Autodesk Inventor part; units mm, degrees
(part 14 of 15)
  line L310 (15.292, -114.284) -> (15.292, -116.316)
  line L311 (15.292, -116.316) -> (16.308, -116.316)
  line L312 (3.408, 49.384) -> (3.408, 51.416)
  line L313 (10.057, -106.5108) -> (10.057, -111.4892)
  line L314 (10.057, -111.4892) -> (12.343, -111.4892)
  line L315 (12.343, -111.4892) -> (12.343, -106.5108)
  line L316 (12.343, -106.5108) -> (10.057, -106.5108)
  line L317 (3.408, 51.416) -> (2.392, 51.416)
  line L318 (1.457, -107.4108) -> (1.457, -112.3892)
  line L319 (1.457, -112.3892) -> (3.743, -112.3892)
  line L320 (3.743, -112.3892) -> (3.743, -107.4108)
  line L321 (3.743, -107.4108) -> (1.457, -107.4108)
  line L322 (2.392, 51.416) -> (2.392, 49.384)
  line L323 (3.765, -108.503) -> (3.765, -111.297)
  line L324 (3.765, -111.297) -> (5.035, -111.297)
  line L325 (5.035, -111.297) -> (5.035, -108.503)
  line L326 (5.035, -108.503) -> (3.765, -108.503)
  line L327 (2.392, 49.384) -> (3.408, 49.384)
  line L328 (8.765, -108.503) -> (8.765, -111.297)
  line L329 (8.765, -111.297) -> (10.035, -111.297)
  line L330 (10.035, -111.297) -> (10.035, -108.503)
  line L331 (10.035, -108.503) -> (8.765, -108.503)
  line L332 (8.616, 35.608) -> (6.584, 35.608)
  line L333 (11.824, -116.313) -> (11.824, -111.487)
  line L334 (11.824, -111.487) -> (8.776, -111.487)
  line L335 (8.776, -111.487) -> (8.776, -116.313)
  line L336 (8.776, -116.313) -> (11.824, -116.313)
  line L337 (6.584, 35.608) -> (6.584, 34.592)
  line L338 (3.776, -100.887) -> (3.776, -105.713)
  line L339 (3.776, -105.713) -> (6.824, -105.713)
  line L340 (6.824, -105.713) -> (6.824, -100.887)
  line L341 (6.824, -100.887) -> (3.776, -100.887)
  line L342 (6.584, 34.592) -> (8.616, 34.592)
  line L343 (16.403, -99.635) -> (19.197, -99.635)
  line L344 (19.197, -99.635) -> (19.197, -98.365)
  line L345 (19.197, -98.365) -> (16.403, -98.365)
  line L346 (16.403, -98.365) -> (16.403, -99.635)
  line L347 (8.616, 34.592) -> (8.616, 35.608)
  line L348 (8.765, -100.903) -> (8.765, -103.697)
  line L349 (8.765, -103.697) -> (10.035, -103.697)
  line L350 (10.035, -103.697) -> (10.035, -100.903)
  line L351 (10.035, -100.903) -> (8.765, -100.903)
  line L352 (8.584, 43.992) -> (10.616, 43.992)
  line L353 (7.165, -100.903) -> (7.165, -103.697)
  line L354 (7.165, -103.697) -> (8.435, -103.697)
  line L355 (8.435, -103.697) -> (8.435, -100.903)
  line L356 (8.435, -100.903) -> (7.165, -100.903)
  line L357 (10.616, 43.992) -> (10.616, 45.008)
  line L358 (-7.387, -104.576) -> (-12.213, -104.576)
  line L359 (-12.213, -104.576) -> (-12.213, -107.624)
  line L360 (-12.213, -107.624) -> (-7.387, -107.624)
  line L361 (-7.387, -107.624) -> (-7.387, -104.576)
  line L362 (10.616, 45.008) -> (8.584, 45.008)
  line L363 (-9.403, -107.965) -> (-12.197, -107.965)
  line L364 (-12.197, -107.965) -> (-12.197, -109.235)
  line L365 (-12.197, -109.235) -> (-9.403, -109.235)
  line L366 (-9.403, -109.235) -> (-9.403, -107.965)
  line L367 (8.584, 45.008) -> (8.584, 43.992)
  line L368 (-4.916, -113.308) -> (-2.884, -113.308)
  line L369 (-2.884, -113.308) -> (-2.884, -112.292)
  line L370 (-2.884, -112.292) -> (-4.916, -112.292)
  line L371 (-4.916, -112.292) -> (-4.916, -113.308)
  line L372 (7.592, 37.616) -> (7.592, 35.584)
  line L373 (11.184, -98.108) -> (13.216, -98.108)
  line L374 (13.216, -98.108) -> (13.216, -97.092)
  line L375 (13.216, -97.092) -> (11.184, -97.092)
  line L376 (11.184, -97.092) -> (11.184, -98.108)
  line L377 (7.592, 35.584) -> (8.608, 35.584)
  line L378 (-7.784, -111.692) -> (-9.816, -111.692)
  line L379 (-9.816, -111.692) -> (-9.816, -112.708)
  line L380 (-9.816, -112.708) -> (-7.784, -112.708)
  line L381 (-7.784, -112.708) -> (-7.784, -111.692)
  line L382 (8.608, 35.584) -> (8.608, 37.616)
  line L383 (17.765, -99.803) -> (17.765, -102.597)
  line L384 (17.765, -102.597) -> (19.035, -102.597)
  line L385 (19.035, -102.597) -> (19.035, -99.803)
  line L386 (19.035, -99.803) -> (17.765, -99.803)
  line L387 (8.608, 37.616) -> (7.592, 37.616)
  line L388 (16.465, -99.803) -> (16.465, -102.597)
  line L389 (16.465, -102.597) -> (17.735, -102.597)
  line L390 (17.735, -102.597) -> (17.735, -99.803)
  line L391 (17.735, -99.803) -> (16.465, -99.803)
  line L392 (7.608, 35.584) -> (7.608, 37.616)
  line L393 (-2.892, -111.316) -> (-2.892, -109.284)
  line L394 (-2.892, -109.284) -> (-3.908, -109.284)
  line L395 (-3.908, -109.284) -> (-3.908, -111.316)
  line L396 (-3.908, -111.316) -> (-2.892, -111.316)
  line L397 (7.608, 37.616) -> (6.592, 37.616)
  line L398 (-9.676, -117.913) -> (-9.676, -113.087)
  line L399 (-9.676, -113.087) -> (-12.724, -113.087)
  line L400 (-12.724, -113.087) -> (-12.724, -117.913)
  line L401 (-12.724, -117.913) -> (-9.676, -117.913)
  line L402 (6.592, 37.616) -> (6.592, 35.584)
  line L403 (3.776, -94.687) -> (3.776, -99.513)
  line L404 (3.776, -99.513) -> (6.824, -99.513)
  line L405 (6.824, -99.513) -> (6.824, -94.687)
  line L406 (6.824, -94.687) -> (3.776, -94.687)
  line L407 (6.592, 35.584) -> (7.608, 35.584)
  line L408 (-8.5892, 45.257) -> (-3.6108, 45.257)
  line L409 (-3.6108, 45.257) -> (-3.6108, 47.543)
  line L410 (-3.6108, 47.543) -> (-8.5892, 47.543)
  line L411 (-8.5892, 47.543) -> (-8.5892, 45.257)
  line L412 (8.608, 45.984) -> (8.608, 48.016)
  line L413 (-9.2892, 36.757) -> (-4.3108, 36.757)
  line L414 (-4.3108, 36.757) -> (-4.3108, 39.043)
  line L415 (-4.3108, 39.043) -> (-9.2892, 39.043)
  line L416 (-9.2892, 39.043) -> (-9.2892, 36.757)
  line L417 (8.608, 48.016) -> (7.592, 48.016)
  line L418 (-4.343, 43.6892) -> (-4.343, 38.7108)
  line L419 (-4.343, 38.7108) -> (-2.057, 38.7108)
  line L420 (-2.057, 38.7108) -> (-2.057, 43.6892)
  line L421 (-2.057, 43.6892) -> (-4.343, 43.6892)
  line L422 (7.592, 48.016) -> (7.592, 45.984)
  line L423 (-6.616, 44.292) -> (-4.584, 44.292)
  line L424 (-4.584, 44.292) -> (-4.584, 45.308)
  line L425 (-4.584, 45.308) -> (-6.616, 45.308)
  line L426 (-6.616, 45.308) -> (-6.616, 44.292)
  line L427 (7.592, 45.984) -> (8.608, 45.984)
  line L428 (0.1542, 45.489) -> (-3.5542, 45.489)
  line L429 (-3.5542, 45.489) -> (-3.5542, 43.711)
  line L430 (-3.5542, 43.711) -> (0.1542, 43.711)
  line L431 (0.1542, 43.711) -> (0.1542, 45.489)
  line L432 (2.308, 43.784) -> (2.308, 45.816)
  line L433 (-2.311, 34.9458) -> (-2.311, 38.6542)
  line L434 (-2.311, 38.6542) -> (-4.089, 38.6542)
  line L435 (-4.089, 38.6542) -> (-4.089, 34.9458)
  line L436 (-4.089, 34.9458) -> (-2.311, 34.9458)
  line L437 (2.308, 45.816) -> (1.292, 45.816)
  line L438 (-3.589, 49.2542) -> (-3.589, 45.5458)
  line L439 (-3.589, 45.5458) -> (-1.811, 45.5458)
  line L440 (-1.811, 45.5458) -> (-1.811, 49.2542)
  line L441 (-1.811, 49.2542) -> (-3.589, 49.2542)
  line L442 (1.292, 45.816) -> (1.292, 43.784)
  line L443 (2.916, -93.492) -> (0.884, -93.492)
  line L444 (0.884, -93.492) -> (0.884, -94.508)
  line L445 (0.884, -94.508) -> (2.916, -94.508)
  line L446 (2.916, -94.508) -> (2.916, -93.492)
  line L447 (1.292, 43.784) -> (2.308, 43.784)
  line L448 (-23.584, -18.692) -> (-25.616, -18.692)
  line L449 (-25.616, -18.692) -> (-25.616, -19.708)
  line L450 (-25.616, -19.708) -> (-23.584, -19.708)
  line L451 (-23.584, -19.708) -> (-23.584, -18.692)
  line L452 (4.316, 44.808) -> (2.284, 44.808)
  line L453 (-23.584, -15.692) -> (-25.616, -15.692)
  line L454 (-25.616, -15.692) -> (-25.616, -16.708)
  line L455 (-25.616, -16.708) -> (-23.584, -16.708)
  line L456 (-23.584, -16.708) -> (-23.584, -15.692)
  line L457 (2.284, 44.808) -> (2.284, 43.792)
  line L458 (-25.608, -16.684) -> (-25.608, -18.716)
  line L459 (-25.608, -18.716) -> (-24.592, -18.716)
  line L460 (-24.592, -18.716) -> (-24.592, -16.684)
  line L461 (-24.592, -16.684) -> (-25.608, -16.684)
  line L462 (2.284, 43.792) -> (4.316, 43.792)
  line L463 (-19.784, -25.192) -> (-21.816, -25.192)
  line L464 (-21.816, -25.192) -> (-21.816, -26.208)
  line L465 (-21.816, -26.208) -> (-19.784, -26.208)
  line L466 (-19.784, -26.208) -> (-19.784, -25.192)
  line L467 (4.316, 43.792) -> (4.316, 44.808)
  line L468 (-22.184, -22.392) -> (-24.216, -22.392)
  line L469 (-24.216, -22.392) -> (-24.216, -23.408)
  line L470 (-24.216, -23.408) -> (-22.184, -23.408)
  line L471 (-22.184, -23.408) -> (-22.184, -22.392)
  line L472 (3.316, 47.008) -> (1.284, 47.008)
  line L473 (-21.808, -19.984) -> (-21.808, -22.016)
  line L474 (-21.808, -22.016) -> (-20.792, -22.016)
  line L475 (-20.792, -22.016) -> (-20.792, -19.984)
  line L476 (-20.792, -19.984) -> (-21.808, -19.984)
  line L477 (1.284, 47.008) -> (1.284, 45.992)
  line L478 (-1.784, -16.092) -> (-3.816, -16.092)
  line L479 (-3.816, -16.092) -> (-3.816, -17.108)
  line L480 (-3.816, -17.108) -> (-1.784, -17.108)
  line L481 (-1.784, -17.108) -> (-1.784, -16.092)
  line L482 (1.284, 45.992) -> (3.316, 45.992)
  line L483 (-7.216, -22.108) -> (-5.184, -22.108)
  line L484 (-5.184, -22.108) -> (-5.184, -21.092)
  line L485 (-5.184, -21.092) -> (-7.216, -21.092)
  line L486 (-7.216, -21.092) -> (-7.216, -22.108)
  line L487 (3.316, 45.992) -> (3.316, 47.008)
  line L488 (-1.784, -15.092) -> (-3.816, -15.092)
  line L489 (-3.816, -15.092) -> (-3.816, -16.108)
  line L490 (-3.816, -16.108) -> (-1.784, -16.108)
  line L491 (-1.784, -16.108) -> (-1.784, -15.092)
  line L492 (1.284, 46.992) -> (3.316, 46.992)
  line L493 (-7.216, -20.108) -> (-5.184, -20.108)
  line L494 (-5.184, -20.108) -> (-5.184, -19.092)
  line L495 (-5.184, -19.092) -> (-7.216, -19.092)
  line L496 (-7.216, -19.092) -> (-7.216, -20.108)
  line L497 (3.316, 46.992) -> (3.316, 48.008)
  line L498 (-7.216, -19.108) -> (-5.184, -19.108)
  line L499 (-5.184, -19.108) -> (-5.184, -18.092)
  line L500 (-5.184, -18.092) -> (-7.216, -18.092)
  line L501 (-7.216, -18.092) -> (-7.216, -19.108)
  line L502 (3.316, 48.008) -> (1.284, 48.008)
  line L503 (-7.216, -17.108) -> (-5.184, -17.108)
  line L504 (-5.184, -17.108) -> (-5.184, -16.092)
  line L505 (-5.184, -16.092) -> (-7.216, -16.092)
  line L506 (-7.216, -16.092) -> (-7.216, -17.108)
  line L507 (1.284, 48.008) -> (1.284, 46.992)
  line L508 (-1.784, -18.092) -> (-3.816, -18.092)
  line L509 (-3.816, -18.092) -> (-3.816, -19.108)
  line L510 (-3.816, -19.108) -> (-1.784, -19.108)
  line L511 (-1.784, -19.108) -> (-1.784, -18.092)
  line L512 (4.316, 39.808) -> (2.284, 39.808)
  line L513 (-7.216, -16.108) -> (-5.184, -16.108)
  line L514 (-5.184, -16.108) -> (-5.184, -15.092)
  line L515 (-5.184, -15.092) -> (-7.216, -15.092)
  line L516 (-7.216, -15.092) -> (-7.216, -16.108)
  line L517 (2.284, 39.808) -> (2.284, 38.792)
  line L518 (-7.216, -23.108) -> (-5.184, -23.108)
  line L519 (-5.184, -23.108) -> (-5.184, -22.092)
  line L520 (-5.184, -22.092) -> (-7.216, -22.092)
  line L521 (-7.216, -22.092) -> (-7.216, -23.108)
  line L522 (2.284, 38.792) -> (4.316, 38.792)
  line L523 (-1.784, -21.092) -> (-3.816, -21.092)
  line L524 (-3.816, -21.092) -> (-3.816, -22.108)
  line L525 (-3.816, -22.108) -> (-1.784, -22.108)
  line L526 (-1.784, -22.108) -> (-1.784, -21.092)
  line L527 (4.316, 38.792) -> (4.316, 39.808)
  line L528 (-1.784, -22.092) -> (-3.816, -22.092)
  line L529 (-3.816, -22.092) -> (-3.816, -23.108)
  line L530 (-3.816, -23.108) -> (-1.784, -23.108)
  line L531 (-1.784, -23.108) -> (-1.784, -22.092)
  line L532 (17.084, -58.708) -> (19.116, -58.708)
  line L533 (-1.784, -19.092) -> (-3.816, -19.092)
  line L534 (-3.816, -19.092) -> (-3.816, -20.108)
  line L535 (-3.816, -20.108) -> (-1.784, -20.108)
  line L536 (-1.784, -20.108) -> (-1.784, -19.092)
  line L537 (19.116, -58.708) -> (19.116, -57.692)
  line L538 (-7.216, -24.108) -> (-5.184, -24.108)
  line L539 (-5.184, -24.108) -> (-5.184, -23.092)
  line L540 (-5.184, -23.092) -> (-7.216, -23.092)
  line L541 (-7.216, -23.092) -> (-7.216, -24.108)
  line L542 (19.116, -57.692) -> (17.084, -57.692)
  line L543 (2.308, -40.816) -> (2.308, -38.784)
  line L544 (2.308, -38.784) -> (1.292, -38.784)
  line L545 (1.292, -38.784) -> (1.292, -40.816)
  line L546 (1.292, -40.816) -> (2.308, -40.816)
  line L547 (17.084, -57.692) -> (17.084, -58.708)
  line L548 (2.284, -38.808) -> (4.316, -38.808)
  line L549 (4.316, -38.808) -> (4.316, -37.792)
  line L550 (4.316, -37.792) -> (2.284, -37.792)
  line L551 (2.284, -37.792) -> (2.284, -38.808)
  line L552 (20.184, -54.908) -> (22.216, -54.908)
  line L553 (-14.316, -41.608) -> (-12.284, -41.608)
  line L554 (-12.284, -41.608) -> (-12.284, -40.592)
  line L555 (-12.284, -40.592) -> (-14.316, -40.592)
  line L556 (-14.316, -40.592) -> (-14.316, -41.608)
  line L557 (22.216, -54.908) -> (22.216, -53.892)
  line L558 (6.208, -40.816) -> (6.208, -38.784)
  line L559 (6.208, -38.784) -> (5.192, -38.784)
  line L560 (5.192, -38.784) -> (5.192, -40.816)
  line L561 (5.192, -40.816) -> (6.208, -40.816)
  line L562 (22.216, -53.892) -> (20.184, -53.892)
  line L563 (6.184, -38.808) -> (8.216, -38.808)
  line L564 (8.216, -38.808) -> (8.216, -37.792)
  line L565 (8.216, -37.792) -> (6.184, -37.792)
  line L566 (6.184, -37.792) -> (6.184, -38.808)
  line L567 (20.184, -53.892) -> (20.184, -54.908)
  line L568 (-5.092, -42.516) -> (-5.092, -40.484)
  line L569 (-5.092, -40.484) -> (-6.108, -40.484)
  line L570 (-6.108, -40.484) -> (-6.108, -42.516)
  line L571 (-6.108, -42.516) -> (-5.092, -42.516)
  line L572 (20.184, -55.908) -> (22.216, -55.908)
  line L573 (21.908, -43.516) -> (21.908, -41.484)
  line L574 (21.908, -41.484) -> (20.892, -41.484)
  line L575 (20.892, -41.484) -> (20.892, -43.516)
  line L576 (20.892, -43.516) -> (21.908, -43.516)
  line L577 (22.216, -55.908) -> (22.216, -54.892)
  line L578 (13.184, -46.208) -> (15.216, -46.208)
  line L579 (15.216, -46.208) -> (15.216, -45.192)
  line L580 (15.216, -45.192) -> (13.184, -45.192)
  line L581 (13.184, -45.192) -> (13.184, -46.208)
  line L582 (22.216, -54.892) -> (20.184, -54.892)
  line L583 (14.092, -48.284) -> (14.092, -50.316)
  line L584 (14.092, -50.316) -> (15.108, -50.316)
  line L585 (15.108, -50.316) -> (15.108, -48.284)
  line L586 (15.108, -48.284) -> (14.092, -48.284)
  line L587 (20.184, -54.892) -> (20.184, -55.908)
  line L588 (17.808, -50.316) -> (17.808, -48.284)
  line L589 (17.808, -48.284) -> (16.792, -48.284)
  line L590 (16.792, -48.284) -> (16.792, -50.316)
  line L591 (16.792, -50.316) -> (17.808, -50.316)
  line L592 (20.184, -56.908) -> (22.216, -56.908)
  line L593 (13.184, -47.208) -> (15.216, -47.208)
  line L594 (15.216, -47.208) -> (15.216, -46.192)
  line L595 (15.216, -46.192) -> (13.184, -46.192)
  line L596 (13.184, -46.192) -> (13.184, -47.208)
  line L597 (22.216, -56.908) -> (22.216, -55.892)
  line L598 (17.216, -46.192) -> (15.184, -46.192)
  line L599 (15.184, -46.192) -> (15.184, -47.208)
  line L600 (15.184, -47.208) -> (17.216, -47.208)
  line L601 (17.216, -47.208) -> (17.216, -46.192)
  line L602 (22.216, -55.892) -> (20.184, -55.892)
  line L603 (4.992, -54.784) -> (4.992, -56.816)
  line L604 (4.992, -56.816) -> (6.008, -56.816)
  line L605 (6.008, -56.816) -> (6.008, -54.784)
  line L606 (6.008, -54.784) -> (4.992, -54.784)
  line L607 (20.184, -55.892) -> (20.184, -56.908)
  line L608 (-3.084, -51.692) -> (-5.116, -51.692)
  line L609 (-5.116, -51.692) -> (-5.116, -52.708)
  line L610 (-5.116, -52.708) -> (-3.084, -52.708)
  line L611 (-3.084, -52.708) -> (-3.084, -51.692)
  line L612 (20.184, -57.908) -> (22.216, -57.908)
  line L613 (-3.084, -48.692) -> (-5.116, -48.692)
  line L614 (-5.116, -48.692) -> (-5.116, -49.708)
  line L615 (-5.116, -49.708) -> (-3.084, -49.708)
  line L616 (-3.084, -49.708) -> (-3.084, -48.692)
  line L617 (22.216, -57.908) -> (22.216, -56.892)
  line L618 (-3.084, -45.692) -> (-5.116, -45.692)
  line L619 (-5.116, -45.692) -> (-5.116, -46.708)
  line L620 (-5.116, -46.708) -> (-3.084, -46.708)
  line L621 (-3.084, -46.708) -> (-3.084, -45.692)
  line L622 (22.216, -56.892) -> (20.184, -56.892)
  line L623 (-3.084, -42.692) -> (-5.116, -42.692)
  line L624 (-5.116, -42.692) -> (-5.116, -43.708)
  line L625 (-5.116, -43.708) -> (-3.084, -43.708)
  line L626 (-3.084, -43.708) -> (-3.084, -42.692)
  line L627 (20.184, -56.892) -> (20.184, -57.908)
  line L628 (5.384, 52.492) -> (7.416, 52.492)
  line L629 (7.416, 52.492) -> (7.416, 53.508)
  line L630 (7.416, 53.508) -> (5.384, 53.508)
  line L631 (5.384, 53.508) -> (5.384, 52.492)
  line L632 (25.316, -56.492) -> (23.284, -56.492)
  line L633 (5.384, 53.492) -> (7.416, 53.492)
  line L634 (7.416, 53.492) -> (7.416, 54.508)
  line L635 (7.416, 54.508) -> (5.384, 54.508)
  line L636 (5.384, 54.508) -> (5.384, 53.492)
  line L637 (23.284, -56.492) -> (23.284, -57.508)
  line L638 (-0.684, 59.708) -> (-2.716, 59.708)
  line L639 (-2.716, 59.708) -> (-2.716, 58.692)
  line L640 (-2.716, 58.692) -> (-0.684, 58.692)
  line L641 (-0.684, 58.692) -> (-0.684, 59.708)
  line L642 (23.284, -57.508) -> (25.316, -57.508)
  line L643 (4.603, 54.565) -> (7.397, 54.565)
  line L644 (7.397, 54.565) -> (7.397, 55.835)
  line L645 (7.397, 55.835) -> (4.603, 55.835)
  line L646 (4.603, 55.835) -> (4.603, 54.565)
  line L647 (25.316, -57.508) -> (25.316, -56.492)
  line L648 (-0.697, 57.665) -> (2.097, 57.665)
  line L649 (2.097, 57.665) -> (2.097, 58.935)
  line L650 (2.097, 58.935) -> (-0.697, 58.935)
  line L651 (-0.697, 58.935) -> (-0.697, 57.665)
  line L652 (25.316, -57.492) -> (23.284, -57.492)
  line L653 (1.616, 54.308) -> (-0.416, 54.308)
  line L654 (-0.416, 54.308) -> (-0.416, 53.292)
  line L655 (-0.416, 53.292) -> (1.616, 53.292)
  line L656 (1.616, 53.292) -> (1.616, 54.308)
  line L657 (23.284, -57.492) -> (23.284, -58.508)
  line L658 (1.616, 53.308) -> (-0.416, 53.308)
  line L659 (-0.416, 53.308) -> (-0.416, 52.292)
  line L660 (-0.416, 52.292) -> (1.616, 52.292)
  line L661 (1.616, 52.292) -> (1.616, 53.308)
  line L662 (23.284, -58.508) -> (25.316, -58.508)
  line L663 (2.397, 52.235) -> (-0.397, 52.235)
  line L664 (-0.397, 52.235) -> (-0.397, 50.965)
  line L665 (-0.397, 50.965) -> (2.397, 50.965)
  line L666 (2.397, 50.965) -> (2.397, 52.235)
  line L667 (25.316, -58.508) -> (25.316, -57.492)
  line L668 (1.616, 57.708) -> (-0.416, 57.708)
  line L669 (-0.416, 57.708) -> (-0.416, 56.692)
  line L670 (-0.416, 56.692) -> (1.616, 56.692)
  line L671 (1.616, 56.692) -> (1.616, 57.708)
  line L672 (41.116, 51.508) -> (39.084, 51.508)
  line L673 (1.616, 56.708) -> (-0.416, 56.708)
  line L674 (-0.416, 56.708) -> (-0.416, 55.692)
  line L675 (-0.416, 55.692) -> (1.616, 55.692)
  line L676 (1.616, 55.692) -> (1.616, 56.708)
  line L677 (39.084, 51.508) -> (39.084, 50.492)
  line L678 (2.397, 55.635) -> (-0.397, 55.635)
  line L679 (-0.397, 55.635) -> (-0.397, 54.365)
  line L680 (-0.397, 54.365) -> (2.397, 54.365)
  line L681 (2.397, 54.365) -> (2.397, 55.635)
  line L682 (39.084, 50.492) -> (41.116, 50.492)
  line L683 (7.416, 51.508) -> (5.384, 51.508)
  line L684 (5.384, 51.508) -> (5.384, 50.492)
  line L685 (5.384, 50.492) -> (7.416, 50.492)
  line L686 (7.416, 50.492) -> (7.416, 51.508)
  line L687 (41.116, 50.492) -> (41.116, 51.508)
  line L688 (-0.584, 54.708) -> (-2.616, 54.708)
  line L689 (-2.616, 54.708) -> (-2.616, 53.692)
  line L690 (-2.616, 53.692) -> (-0.584, 53.692)
  line L691 (-0.584, 53.692) -> (-0.584, 54.708)
  line L692 (41.116, 50.508) -> (39.084, 50.508)
  line L693 (-0.584, 56.708) -> (-2.616, 56.708)
  line L694 (-2.616, 56.708) -> (-2.616, 55.692)
  line L695 (-2.616, 55.692) -> (-0.584, 55.692)
  line L696 (-0.584, 55.692) -> (-0.584, 56.708)
  line L697 (39.084, 50.508) -> (39.084, 49.492)
  line L698 (7.416, 52.508) -> (5.384, 52.508)
  line L699 (5.384, 52.508) -> (5.384, 51.492)
  line L700 (5.384, 51.492) -> (7.416, 51.492)
  line L701 (7.416, 51.492) -> (7.416, 52.508)
  line L702 (39.084, 49.492) -> (41.116, 49.492)
  line L703 (-0.584, 53.708) -> (-2.616, 53.708)
  line L704 (-2.616, 53.708) -> (-2.616, 52.692)
  line L705 (-2.616, 52.692) -> (-0.584, 52.692)
  line L706 (-0.584, 52.692) -> (-0.584, 53.708)
  line L707 (41.116, 49.492) -> (41.116, 50.508)
  line L708 (-0.584, 55.708) -> (-2.616, 55.708)
  line L709 (-2.616, 55.708) -> (-2.616, 54.692)
  line L710 (-2.616, 54.692) -> (-0.584, 54.692)
  line L711 (-0.584, 54.692) -> (-0.584, 55.708)
  line L712 (41.116, 49.508) -> (39.084, 49.508)
  line L713 (4.584, 34.592) -> (6.616, 34.592)
  line L714 (6.616, 34.592) -> (6.616, 35.608)
  line L715 (6.616, 35.608) -> (4.584, 35.608)
  line L716 (4.584, 35.608) -> (4.584, 34.592)
  line L717 (39.084, 49.508) -> (39.084, 48.492)
  line L718 (8.584, 42.992) -> (10.616, 42.992)
  line L719 (10.616, 42.992) -> (10.616, 44.008)
  line L720 (10.616, 44.008) -> (8.584, 44.008)
  line L721 (8.584, 44.008) -> (8.584, 42.992)
  line L722 (39.084, 48.492) -> (41.116, 48.492)
  line L723 (8.584, 41.992) -> (10.616, 41.992)
  line L724 (10.616, 41.992) -> (10.616, 43.008)
  line L725 (10.616, 43.008) -> (8.584, 43.008)
  line L726 (8.584, 43.008) -> (8.584, 41.992)
  line L727 (41.116, 48.492) -> (41.116, 49.508)
  line L728 (1.292, 43.816) -> (1.292, 41.784)
  line L729 (1.292, 41.784) -> (2.308, 41.784)
  line L730 (2.308, 41.784) -> (2.308, 43.816)
  line L731 (2.308, 43.816) -> (1.292, 43.816)
  line L732 (41.116, 48.508) -> (39.084, 48.508)
  line L733 (2.308, 39.784) -> (2.308, 41.816)
  line L734 (2.308, 41.816) -> (1.292, 41.816)
  line L735 (1.292, 41.816) -> (1.292, 39.784)
  line L736 (1.292, 39.784) -> (2.308, 39.784)
  line L737 (39.084, 48.508) -> (39.084, 47.492)
  line L738 (7.608, 45.984) -> (7.608, 48.016)
  line L739 (7.608, 48.016) -> (6.592, 48.016)
  line L740 (6.592, 48.016) -> (6.592, 45.984)
  line L741 (6.592, 45.984) -> (7.608, 45.984)
  line L742 (39.084, 47.492) -> (41.116, 47.492)
  line L743 (6.585, 46.003) -> (6.585, 48.797)
  line L744 (6.585, 48.797) -> (5.315, 48.797)
  line L745 (5.315, 48.797) -> (5.315, 46.003)
  line L746 (5.315, 46.003) -> (6.585, 46.003)
  line L747 (41.116, 47.492) -> (41.116, 48.508)
  line L748 (4.292, 48.016) -> (4.292, 45.984)
  line L749 (4.292, 45.984) -> (5.308, 45.984)
  line L750 (5.308, 45.984) -> (5.308, 48.016)
  line L751 (5.308, 48.016) -> (4.292, 48.016)
  line L752 (41.116, 44.008) -> (39.084, 44.008)
  line L753 (3.292, 48.016) -> (3.292, 45.984)
  line L754 (3.292, 45.984) -> (4.308, 45.984)
  line L755 (4.308, 45.984) -> (4.308, 48.016)
  line L756 (4.308, 48.016) -> (3.292, 48.016)
  line L757 (39.084, 44.008) -> (39.084, 42.992)
  line L758 (6.608, 35.584) -> (6.608, 37.616)
  line L759 (6.608, 37.616) -> (5.592, 37.616)
  line L760 (5.592, 37.616) -> (5.592, 35.584)
  line L761 (5.592, 35.584) -> (6.608, 35.584)
  line L762 (39.084, 42.992) -> (41.116, 42.992)
  line L763 (5.608, 35.584) -> (5.608, 37.616)
  line L764 (5.608, 37.616) -> (4.592, 37.616)
  line L765 (4.592, 37.616) -> (4.592, 35.584)
  line L766 (4.592, 35.584) -> (5.608, 35.584)
  line L767 (41.116, 42.992) -> (41.116, 44.008)
  line L768 (5.608, 37.584) -> (5.608, 39.616)
  line L769 (5.608, 39.616) -> (4.592, 39.616)
  line L770 (4.592, 39.616) -> (4.592, 37.584)
  line L771 (4.592, 37.584) -> (5.608, 37.584)
  line L772 (-23.116, -27.908) -> (-21.084, -27.908)
  line L773 (2.284, 42.792) -> (4.316, 42.792)
  line L774 (4.316, 42.792) -> (4.316, 43.808)
  line L775 (4.316, 43.808) -> (2.284, 43.808)
  line L776 (2.284, 43.808) -> (2.284, 42.792)
  line L777 (-21.084, -27.908) -> (-21.084, -26.892)
  line L778 (4.592, 46.016) -> (4.592, 43.984)
  line L779 (4.592, 43.984) -> (5.608, 43.984)
  line L780 (5.608, 43.984) -> (5.608, 46.016)
  line L781 (5.608, 46.016) -> (4.592, 46.016)
  line L782 (-21.084, -26.892) -> (-23.116, -26.892)
  line L783 (6.608, 37.584) -> (6.608, 39.616)
  line L784 (6.608, 39.616) -> (5.592, 39.616)
  line L785 (5.592, 39.616) -> (5.592, 37.584)
  line L786 (5.592, 37.584) -> (6.608, 37.584)
  line L787 (-23.116, -26.892) -> (-23.116, -27.908)
  line L788 (2.284, 41.792) -> (4.316, 41.792)
  line L789 (4.316, 41.792) -> (4.316, 42.808)
  line L790 (4.316, 42.808) -> (2.284, 42.808)
  line L791 (2.284, 42.808) -> (2.284, 41.792)
  line L792 (-23.284, -26.892) -> (-25.316, -26.892)
  line L793 (5.592, 46.016) -> (5.592, 43.984)
  line L794 (5.592, 43.984) -> (6.608, 43.984)
  line L795 (6.608, 43.984) -> (6.608, 46.016)
  line L796 (6.608, 46.016) -> (5.592, 46.016)
  line L797 (-25.316, -26.892) -> (-25.316, -27.908)
  line L798 (7.608, 37.584) -> (7.608, 39.616)
  line L799 (7.608, 39.616) -> (6.592, 39.616)
  line L800 (6.592, 39.616) -> (6.592, 37.584)
  line L801 (6.592, 37.584) -> (7.608, 37.584)
  line L802 (-25.316, -27.908) -> (-23.284, -27.908)
  line L803 (10.616, 41.608) -> (8.584, 41.608)
  line L804 (8.584, 41.608) -> (8.584, 40.592)
  line L805 (8.584, 40.592) -> (10.616, 40.592)
  line L806 (10.616, 40.592) -> (10.616, 41.608)
  line L807 (-23.284, -27.908) -> (-23.284, -26.892)
  line L808 (2.284, 40.792) -> (4.316, 40.792)
  line L809 (4.316, 40.792) -> (4.316, 41.808)
  line L810 (4.316, 41.808) -> (2.284, 41.808)
  line L811 (2.284, 41.808) -> (2.284, 40.792)
  line L812 (6.5, -90.25) -> (6.5, -91.34)
  line L813 (6.592, 46.016) -> (6.592, 43.984)
  line L814 (6.592, 43.984) -> (7.608, 43.984)
  line L815 (7.608, 43.984) -> (7.608, 46.016)
  line L816 (7.608, 46.016) -> (6.592, 46.016)
  line L817 (9.7, -90.05) -> (6.5, -90.05)
  line L818 (8.608, 37.584) -> (8.608, 39.616)
  line L819 (8.608, 39.616) -> (7.592, 39.616)
  line L820 (7.592, 39.616) -> (7.592, 37.584)
  line L821 (7.592, 37.584) -> (8.608, 37.584)
  line L822 (6.5, -90.05) -> (6.5, -91.55)
  line L823 (10.616, 40.608) -> (8.584, 40.608)
  line L824 (8.584, 40.608) -> (8.584, 39.592)
  line L825 (8.584, 39.592) -> (10.616, 39.592)
  line L826 (10.616, 39.592) -> (10.616, 40.608)
  line L827 (6.5, -91.55) -> (9.7, -91.55)
  line L828 (2.284, 39.792) -> (4.316, 39.792)
  line L829 (4.316, 39.792) -> (4.316, 40.808)
  line L830 (4.316, 40.808) -> (2.284, 40.808)
  line L831 (2.284, 40.808) -> (2.284, 39.792)
  line L832 (9.7, -91.55) -> (9.7, -90.05)
  line L833 (7.592, 46.016) -> (7.592, 43.984)
  line L834 (7.592, 43.984) -> (8.608, 43.984)
  line L835 (8.608, 43.984) -> (8.608, 46.016)
  line L836 (8.608, 46.016) -> (7.592, 46.016)
  circle A125 centre (9.29, -90.4) radius 0.15
  line L837 (18.608, -54.516) -> (18.608, -52.484)
  line L838 (18.608, -52.484) -> (17.592, -52.484)
  line L839 (17.592, -52.484) -> (17.592, -54.516)
  line L840 (17.592, -54.516) -> (18.608, -54.516)
  line L841 (2.05, -44.95) -> (5.15, -44.95)
  line L842 (23.284, -54.908) -> (25.316, -54.908)
  line L843 (25.316, -54.908) -> (25.316, -53.892)
  line L844 (25.316, -53.892) -> (23.284, -53.892)
  line L845 (23.284, -53.892) -> (23.284, -54.908)
  line L846 (5.15, -44.95) -> (5.15, -42.45)
  line L847 (-1.784, -20.092) -> (-3.816, -20.092)
  line L848 (-3.816, -20.092) -> (-3.816, -21.108)
  line L849 (-3.816, -21.108) -> (-1.784, -21.108)
  line L850 (-1.784, -21.108) -> (-1.784, -20.092)
  line L851 (5.15, -42.45) -> (2.05, -42.45)
  line L852 (-7.216, -18.108) -> (-5.184, -18.108)
  line L853 (-5.184, -18.108) -> (-5.184, -17.092)
  line L854 (-5.184, -17.092) -> (-7.216, -17.092)
  line L855 (-7.216, -17.092) -> (-7.216, -18.108)
  line L856 (2.05, -42.45) -> (2.05, -44.95)
  line L857 (-7.216, -21.108) -> (-5.184, -21.108)
  line L858 (-5.184, -21.108) -> (-5.184, -20.092)
  line L859 (-5.184, -20.092) -> (-7.216, -20.092)
  line L860 (-7.216, -20.092) -> (-7.216, -21.108)
  circle A126 centre (2.8, -43.1) radius 0.1
  line L861 (-1.784, -17.092) -> (-3.816, -17.092)
  line L862 (-3.816, -17.092) -> (-3.816, -18.108)
  line L863 (-3.816, -18.108) -> (-1.784, -18.108)
  line L864 (-1.784, -18.108) -> (-1.784, -17.092)
  line L865 (-20.584, -109.492) -> (-22.616, -109.492)
  line L866 (-22.616, -109.492) -> (-22.616, -110.508)
  line L867 (-22.616, -110.508) -> (-20.584, -110.508)
  line L868 (-20.584, -110.508) -> (-20.584, -109.492)
  line L869 (14.924, -116.313) -> (14.924, -111.487)
  line L870 (14.924, -111.487) -> (11.876, -111.487)
  line L871 (11.876, -111.487) -> (11.876, -116.313)
  line L872 (11.876, -116.313) -> (14.924, -116.313)
  line L873 (-47.3, -31.385) -> (-48.9, -31.385)
  circle A127 centre (-48.1, -47.7) radius 15.9
  line L874 (-16.5514, 47.555) -> (-16.5514, 47.255)
  line L875 (-16.5514, 46.455) -> (-16.5514, 46.155)
  line L876 (-16.5514, 45.355) -> (-16.5514, 45.055)
  line L877 (-16.5514, 44.255) -> (-16.5514, 43.955)
  line L878 (-16.5514, 43.155) -> (-16.5514, 42.855)
  line L879 (-16.5514, 42.055) -> (-16.5514, 41.755)
  line L880 (-16.5514, 40.955) -> (-16.5514, 40.655)
  line L881 (-16.5514, 39.855) -> (-16.5514, 39.555)
  line L882 (-22.4, 38.105) -> (-22.4, 37.385)
  line L883 (-15.05, 47.655) -> (-15.05, 39.105)
  arc A128 (-15.3, 38.855) -> (-15.05, 39.105) centre (-15.3, 39.105) ccw
  line L884 (-15.3, 38.855) -> (-16.3, 38.855)
  arc A129 (-16.55, 39.105) -> (-16.3, 38.855) centre (-16.3, 39.105) ccw
  line L885 (-16.55, 39.105) -> (-16.55, 47.655)
  arc A130 (-16.3, 47.905) -> (-16.55, 47.655) centre (-16.3, 47.655) ccw
  line L886 (-16.3, 47.905) -> (-15.3, 47.905)
  arc A131 (-15.05, 47.655) -> (-15.3, 47.905) centre (-15.3, 47.655) ccw
  line L887 (-24.45, 36.285) -> (-24.45, 36.105)
  line L888 (-24.45, 36.105) -> (-22.4, 36.105)
  line L889 (-22.4, 36.105) -> (-21.195, 36.105)
  line L890 (-21.195, 36.105) -> (-14.305, 36.105)
  line L891 (-14.305, 36.105) -> (-12.895, 36.105)
  line L892 (-12.895, 36.105) -> (-11.05, 36.105)
  line L893 (-11.05, 36.105) -> (-11.05, 37.155)
  line L894 (-11.05, 37.155) -> (-11.7948, 37.4261)
  arc A132 (-12.1166, 37.8115) -> (-11.7948, 37.4262) centre (-11.6238, 37.896) ccw
  arc A133 (-12.1167, 47.9985) -> (-12.1167, 37.8115) centre (17.6036, 42.905) ccw
  line L895 (-22.68, 36.295) -> (-25.5, 36.295)
  arc A134 (-25.55, 36.345) -> (-25.5, 36.295) centre (-25.5, 36.345) ccw
  line L896 (-25.55, 36.345) -> (-25.55, 36.805)
  arc A135 (-25.5, 36.855) -> (-25.55, 36.805) centre (-25.5, 36.805) ccw
  arc A136 (-25.55, 49.005) -> (-25.5, 48.955) centre (-25.5, 49.005) ccw
  line L897 (-25.55, 49.005) -> (-25.55, 49.465)
  arc A137 (-25.5, 49.515) -> (-25.55, 49.465) centre (-25.5, 49.465) ccw
  line L898 (-25.5, 49.515) -> (-22.68, 49.515)
  line L899 (-11.05, 48.655) -> (-11.05, 49.705)
  line L900 (-11.05, 49.705) -> (-12.895, 49.705)
  line L901 (-12.895, 49.705) -> (-14.305, 49.705)
  line L902 (-14.305, 49.705) -> (-21.195, 49.705)
  line L903 (-21.195, 49.705) -> (-22.4, 49.705)
  line L904 (-22.4, 49.705) -> (-24.45, 49.705)
  line L905 (-24.45, 49.705) -> (-24.45, 49.525)
  line L906 (-22.4, 36.105) -> (-22.4, 38.4841)
  line L907 (-22.4, 38.4841) -> (-22.4, 38.755)
  arc A138 (-22.4, 38.755) -> (-22.4, 38.955) centre (-22.4, 38.855) ccw
  line L908 (-22.4, 38.955) -> (-22.4, 39.305)
  arc A139 (-22.4, 39.305) -> (-22.4, 39.505) centre (-22.4, 39.405) ccw
  line L909 (-22.4, 39.505) -> (-22.4, 46.305)
  arc A140 (-22.4, 46.305) -> (-22.4, 46.505) centre (-22.4, 46.405) ccw
  line L910 (-22.4, 46.505) -> (-22.4, 46.855)
  arc A141 (-22.4, 46.855) -> (-22.4, 47.055) centre (-22.4, 46.955) ccw
  line L911 (-22.4, 47.055) -> (-22.4, 49.705)
  line L912 (-25.55, 38.4841) -> (-22.4, 38.4841)
  line L913 (-12.895, 49.705) -> (-12.895, 50.125)
  arc A142 (-12.895, 50.125) -> (-12.975, 50.205) centre (-12.975, 50.125) ccw
  line L914 (-12.975, 50.205) -> (-13.225, 50.205)
  line L915 (-13.225, 50.205) -> (-13.35, 50.085)
  line L916 (-13.35, 50.085) -> (-13.85, 50.085)
  line L917 (-13.85, 50.085) -> (-13.975, 50.205)
  line L918 (-13.975, 50.205) -> (-14.225, 50.205)
  arc A143 (-14.225, 50.205) -> (-14.305, 50.125) centre (-14.225, 50.125) ccw
  line L919 (-14.305, 50.125) -> (-14.305, 49.705)
  line L920 (-21.195, 49.705) -> (-21.195, 50.125)
  arc A144 (-21.195, 50.125) -> (-21.275, 50.205) centre (-21.275, 50.125) ccw
  line L921 (-21.275, 50.205) -> (-21.525, 50.205)
  line L922 (-21.525, 50.205) -> (-21.65, 50.085)
  line L923 (-21.65, 50.085) -> (-22.15, 50.085)
  line L924 (-22.15, 50.085) -> (-22.275, 50.205)
  line L925 (-22.275, 50.205) -> (-22.525, 50.205)
  arc A145 (-22.525, 50.205) -> (-22.605, 50.125) centre (-22.525, 50.125) ccw
  line L926 (-22.605, 50.125) -> (-22.605, 49.455)
  line L927 (-22.605, 49.455) -> (-22.6, 49.455)
  line L928 (-22.6, 49.455) -> (-22.6, 48.955)
  line L929 (-22.6, 48.955) -> (-23.1, 48.955)
  line L930 (-23.1, 48.955) -> (-23.1, 49.105)
  line L931 (-23.1, 49.105) -> (-22.85, 49.105)
  line L932 (-22.85, 49.105) -> (-22.8, 49.155)
  line L933 (-22.8, 49.155) -> (-22.8, 49.305)
  line L934 (-22.8, 49.305) -> (-22.85, 49.355)
  line L935 (-22.85, 49.355) -> (-25.3, 49.355)
  line L936 (-25.3, 49.355) -> (-25.35, 49.305)
  line L937 (-25.35, 49.305) -> (-25.35, 49.155)
  line L938 (-25.35, 49.155) -> (-25.3, 49.105)
  line L939 (-25.3, 49.105) -> (-25.05, 49.105)
  line L940 (-25.05, 49.105) -> (-25.05, 48.955)
  line L941 (-25.05, 48.955) -> (-25.55, 48.955)
  line L942 (-25.55, 48.955) -> (-25.55, 38.4841)
  line L943 (-25.55, 38.4841) -> (-25.55, 36.855)
  line L944 (-25.55, 36.855) -> (-25.05, 36.855)
  line L945 (-25.05, 36.855) -> (-25.05, 36.705)
  line L946 (-25.05, 36.705) -> (-25.3, 36.705)
  line L947 (-25.3, 36.705) -> (-25.35, 36.655)
  line L948 (-25.35, 36.655) -> (-25.35, 36.505)
  line L949 (-25.35, 36.505) -> (-25.3, 36.455)
  line L950 (-25.3, 36.455) -> (-22.85, 36.455)
  line L951 (-22.85, 36.455) -> (-22.8, 36.505)
  line L952 (-22.8, 36.505) -> (-22.8, 36.655)
  line L953 (-22.8, 36.655) -> (-22.85, 36.705)
  line L954 (-22.85, 36.705) -> (-23.1, 36.705)
  line L955 (-23.1, 36.705) -> (-23.1, 36.855)
  line L956 (-23.1, 36.855) -> (-22.6, 36.855)
  line L957 (-22.6, 36.855) -> (-22.6, 36.355)
  line L958 (-22.6, 36.355) -> (-22.605, 36.355)
  line L959 (-22.605, 36.355) -> (-22.605, 35.685)
  arc A146 (-22.605, 35.685) -> (-22.525, 35.605) centre (-22.525, 35.685) ccw
  line L960 (-22.525, 35.605) -> (-22.275, 35.605)
  line L961 (-22.275, 35.605) -> (-22.15, 35.725)
  line L962 (-22.15, 35.725) -> (-21.65, 35.725)
  line L963 (-21.65, 35.725) -> (-21.525, 35.605)
  line L964 (-21.525, 35.605) -> (-21.275, 35.605)
  arc A147 (-21.275, 35.605) -> (-21.195, 35.685) centre (-21.275, 35.685) ccw
  line L965 (-21.195, 35.685) -> (-21.195, 36.105)
  line L966 (-14.305, 36.105) -> (-14.305, 35.685)
  arc A148 (-14.305, 35.685) -> (-14.225, 35.605) centre (-14.225, 35.685) ccw
  line L967 (-14.225, 35.605) -> (-13.975, 35.605)
  line L968 (-13.975, 35.605) -> (-13.85, 35.725)
  line L969 (-13.85, 35.725) -> (-13.35, 35.725)
  line L970 (-13.35, 35.725) -> (-13.225, 35.605)
  line L971 (-13.225, 35.605) -> (-12.975, 35.605)
  arc A149 (-12.975, 35.605) -> (-12.895, 35.685) centre (-12.975, 35.685) ccw
  line L972 (-12.895, 35.685) -> (-12.895, 36.105)
  arc A150 (-11.7948, 48.3838) -> (-12.1166, 47.9985) centre (-11.6238, 47.914) ccw
  arc A151 (-11.7948, 48.3838) -> (-12.1166, 47.9985) centre (-11.6238, 47.914) ccw
  line L973 (-11.7948, 48.3839) -> (-11.05, 48.655)
  line L974 (65.55, 33.9) -> (70.05, 33.9)
  line L975 (70.05, 33.9) -> (70.05, 55.3)
  line L976 (70.05, 55.3) -> (65.55, 55.3)
  line L977 (65.55, 55.3) -> (65.55, 33.9)
  line L978 (66.3, 53.6) -> (67.3, 54.1)
  line L979 (66.3, 54.6) -> (66.3, 53.6)
  line L980 (67.3, 54.1) -> (66.3, 54.6)
  line L981 (22.55, -102.1) -> (25.05, -102.1)
  line L982 (25.05, -101.1) -> (22.55, -101.1)
  line L983 (25.05, -102.1) -> (25.05, -101.1)
  line L984 (22.55, -101.1) -> (22.55, -102.1)
  circle A152 centre (24.7, -101.8) radius 0.05
  line L985 (22.15, -101.1) -> (19.65, -101.1)
  line L986 (19.65, -102.1) -> (22.15, -102.1)
  line L987 (19.65, -101.1) -> (19.65, -102.1)
  line L988 (22.15, -102.1) -> (22.15, -101.1)
  circle A153 centre (20, -101.4) radius 0.05
  line L989 (-18.8, -16.95) -> (-18.8, -19.45)
  line L990 (-17.8, -19.45) -> (-17.8, -16.95)
  line L991 (-18.8, -19.45) -> (-17.8, -19.45)
  line L992 (-17.8, -16.95) -> (-18.8, -16.95)
  circle A154 centre (-18.5, -19.1) radius 0.05
  line L993 (-17.8, -16.65) -> (-17.8, -14.15)
  line L994 (-18.8, -14.15) -> (-18.8, -16.65)
  line L995 (-17.8, -14.15) -> (-18.8, -14.15)
  line L996 (-18.8, -16.65) -> (-17.8, -16.65)
  circle A155 centre (-18.1, -14.5) radius 0.05
  line L997 (22.05, -44.5) -> (19.55, -44.5)
  line L998 (19.55, -45.5) -> (22.05, -45.5)
  line L999 (19.55, -44.5) -> (19.55, -45.5)
  line L1000 (22.05, -45.5) -> (22.05, -44.5)
  circle A156 centre (19.9, -44.8) radius 0.05
  line L1001 (22.35, -45.5) -> (24.85, -45.5)
  line L1002 (24.85, -44.5) -> (22.35, -44.5)
  line L1003 (24.85, -45.5) -> (24.85, -44.5)
  line L1004 (22.35, -44.5) -> (22.35, -45.5)
  circle A157 centre (24.5, -45.2) radius 0.05
  line L1005 (0, -50.05) -> (0, -52.55)
  line L1006 (1, -52.55) -> (1, -50.05)
  line L1007 (0, -52.55) -> (1, -52.55)
  line L1008 (1, -50.05) -> (0, -50.05)
  circle A158 centre (0.3, -52.2) radius 0.05
  line L1009 (0, -47.05) -> (0, -49.55)
  line L1010 (1, -49.55) -> (1, -47.05)
  line L1011 (0, -49.55) -> (1, -49.55)
  line L1012 (1, -47.05) -> (0, -47.05)
  circle A159 centre (0.3, -49.2) radius 0.05
  line L1013 (7.3542, 50.489) -> (5.0458, 50.489)
  line L1014 (5.0458, 50.489) -> (5.0458, 49.511)
  line L1015 (5.0458, 49.511) -> (7.3542, 49.511)
  line L1016 (7.3542, 49.511) -> (7.3542, 50.489)
  line L1017 (-0.4458, 51.989) -> (-2.7542, 51.989)
  line L1018 (-2.7542, 51.989) -> (-2.7542, 51.011)
  line L1019 (-2.7542, 51.011) -> (-0.4458, 51.011)
  line L1020 (-0.4458, 51.011) -> (-0.4458, 51.989)
  line L1021 (-0.5458, 57.689) -> (-2.8542, 57.689)
  line L1022 (-2.8542, 57.689) -> (-2.8542, 56.711)
  line L1023 (-2.8542, 56.711) -> (-0.5458, 56.711)
  line L1024 (-0.5458, 56.711) -> (-0.5458, 57.689)
  line L1025 (3.511, 38.5542) -> (3.511, 36.2458)
  line L1026 (3.511, 36.2458) -> (4.489, 36.2458)
  line L1027 (4.489, 36.2458) -> (4.489, 38.5542)
  line L1028 (4.489, 38.5542) -> (3.511, 38.5542)
  line L1029 (9.211, 39.5542) -> (9.211, 37.2458)
  line L1030 (9.211, 37.2458) -> (10.189, 37.2458)
  line L1031 (10.189, 37.2458) -> (10.189, 39.5542)
  line L1032 (10.189, 39.5542) -> (9.211, 39.5542)
  line L1033 (2.311, 38.5542) -> (2.311, 36.2458)
  line L1034 (2.311, 36.2458) -> (3.289, 36.2458)
  line L1035 (3.289, 36.2458) -> (3.289, 38.5542)
  line L1036 (3.289, 38.5542) -> (2.311, 38.5542)
  line L1037 (4.5542, 45.889) -> (2.2458, 45.889)
  line L1038 (2.2458, 45.889) -> (2.2458, 44.911)
  line L1039 (2.2458, 44.911) -> (4.5542, 44.911)
  line L1040 (4.5542, 44.911) -> (4.5542, 45.889)
  line L1041 (-19.5, -107.4) -> (-19.5, -110.4)
  line L1042 (-16.5, -110.4) -> (-16.5, -107.4)
  line L1043 (-16.5, -107.4) -> (-19.5, -107.4)
  line L1044 (-19.5, -110.4) -> (-16.5, -110.4)
  circle A160 centre (-19.18, -107.72) radius 0.05
  line L1045 (7.9, -78.7) -> (7.9, -86.7)
  line L1046 (15.9, -86.7) -> (15.9, -78.7)
  line L1047 (15.9, -78.7) -> (7.9, -78.7)
  line L1048 (7.9, -86.7) -> (15.9, -86.7)
  circle A161 centre (8.5, -79.4) radius 0.2828
  line L1049 (16.6, -115) -> (19.6, -115)
  line L1050 (19.6, -112) -> (16.6, -112)
  line L1051 (16.6, -112) -> (16.6, -115)
  line L1052 (19.6, -115) -> (19.6, -112)
  circle A162 centre (17.1, -112.4) radius 0.1414
  line L1053 (8.075, -107.225) -> (5.525, -107.225)
  line L1054 (5.525, -107.225) -> (5.525, -110.775)
  line L1055 (5.525, -110.775) -> (8.075, -110.775)
  line L1056 (8.075, -110.775) -> (8.075, -107.225)
  circle A163 centre (7.7, -107.6) radius 0.1414
  line L1057 (11.4, -98.5) -> (11.4, -102.5)
  line L1058 (15.4, -102.5) -> (15.4, -98.5)
  line L1059 (15.4, -98.5) -> (11.4, -98.5)
  line L1060 (11.4, -102.5) -> (15.4, -102.5)
  circle A164 centre (11.72, -98.82) radius 0.05
  line L1061 (-9, -108.2) -> (-9, -111.2)
  line L1062 (-6, -111.2) -> (-6, -108.2)
  line L1063 (-6, -108.2) -> (-9, -108.2)
  line L1064 (-9, -111.2) -> (-6, -111.2)
  circle A165 centre (-8.68, -108.52) radius 0.05
  line L1065 (-8.9, 43.8) -> (-8.9, 39.8)
  line L1066 (-8.9, 39.8) -> (-4.9, 39.8)
  line L1067 (-4.9, 39.8) -> (-4.9, 43.8)
  line L1068 (-4.9, 43.8) -> (-8.9, 43.8)
  circle A166 centre (-8.5, 40.2) radius 0.2236
  line L1069 (2.9, -89) -> (-0.1, -89)
  line L1070 (-0.1, -92) -> (2.9, -92)
  line L1071 (2.9, -92) -> (2.9, -89)
  line L1072 (-0.1, -89) -> (-0.1, -92)
  circle A167 centre (2.5, -91.6) radius 0.1414
  line L1073 (11.5, -13.3) -> (11.5, -1.55)
  line L1074 (11.5, -13.3) -> (-0.25, -13.3)
  line L1075 (11.5, 21.7) -> (11.5, 13.95)
  line L1076 (11.5, 21.7) -> (-0.25, 21.7)
  line L1077 (-23.5, 21.7) -> (-23.5, 13.95)
  line L1078 (-23.5, 21.7) -> (-15.75, 21.7)
  line L1079 (-23.5, -13.3) -> (-23.5, -1.55)
  line L1080 (-23.5, -13.3) -> (-15.75, -13.3)
  circle A168 centre (-22.5, 22.2) radius 0.1
  line L1081 (-17.4332, -25.6112) -> (-19.5668, -25.6112)
  line L1082 (-19.5668, -25.6112) -> (-19.5668, -25.2048)
  line L1083 (-19.5668, -25.2048) -> (-19.5668, -25.1286)
  line L1084 (-19.5668, -25.1286) -> (-19.5668, -24.6714)
  line L1085 (-19.5668, -24.6714) -> (-19.5668, -24.5952)
  line L1086 (-19.5668, -24.5952) -> (-19.5668, -24.1888)
  arc A169 (-19.5668, -25.2048) -> (-19.5668, -24.5952) centre (-19.5668, -24.9) ccw
  line L1087 (-17.4332, -24.6714) -> (-17.4332, -25.1286)
  line L1088 (-18.373, -25.6112) -> (-18.627, -25.6112)
  line L1089 (-19.5668, -25.1286) -> (-19.5668, -24.6714)
  line L1090 (-17.4332, -24.1888) -> (-17.4332, -25.6112)
  line L1091 (-19.5668, -24.1888) -> (-17.4332, -24.1888)
  line L1092 (25.3, 21.7) -> (25.3, 11.7)
  line L1093 (25.3, 11.7) -> (12.3, 11.7)
  line L1094 (12.3, 11.7) -> (12.3, 21.7)
  line L1095 (12.3, 21.7) -> (25.3, 21.7)
  line L1096 (12.5, 21) -> (13, 21.5)
  line L1097 (12.5, 21.5) -> (12.5, 21)
  line L1098 (13, 21.5) -> (12.5, 21.5)
  line L1099 (25.3, 11.3) -> (25.3, 1.3)
  line L1100 (25.3, 1.3) -> (12.3, 1.3)
  line L1101 (12.3, 1.3) -> (12.3, 11.3)
  line L1102 (12.3, 11.3) -> (25.3, 11.3)
  line L1103 (12.5, 10.6) -> (13, 11.1)
  line L1104 (12.5, 11.1) -> (12.5, 10.6)
  line L1105 (13, 11.1) -> (12.5, 11.1)
  line L1106 (25.3, 0.9) -> (25.3, -9.1)
  line L1107 (25.3, -9.1) -> (12.3, -9.1)
  line L1108 (12.3, -9.1) -> (12.3, 0.9)
  line L1109 (12.3, 0.9) -> (25.3, 0.9)
  line L1110 (12.5, 0.2) -> (13, 0.7)
  line L1111 (12.5, 0.7) -> (12.5, 0.2)
  line L1112 (13, 0.7) -> (12.5, 0.7)
  line L1113 (25.3, -9.5) -> (25.3, -19.5)
  line L1114 (25.3, -19.5) -> (12.3, -19.5)
  line L1115 (12.3, -19.5) -> (12.3, -9.5)
  line L1116 (12.3, -9.5) -> (25.3, -9.5)
  line L1117 (12.5, -10.2) -> (13, -9.7)
  line L1118 (12.5, -9.7) -> (12.5, -10.2)
  line L1119 (13, -9.7) -> (12.5, -9.7)
  line L1120 (-1.5, -24.3) -> (-1.5, -14.3)
  line L1121 (-1.5, -14.3) -> (11.5, -14.3)
  line L1122 (11.5, -14.3) -> (11.5, -24.3)
  line L1123 (11.5, -24.3) -> (-1.5, -24.3)
  line L1124 (11.3, -23.6) -> (10.8, -24.1)
  line L1125 (11.3, -24.1) -> (11.3, -23.6)
  line L1126 (10.8, -24.1) -> (11.3, -24.1)
  line L1127 (2.5662, -52.6496) -> (2.5662, -53.2338)
  line L1128 (2.5662, -53.2338) -> (3.1504, -53.2338)
  line L1129 (9.729, -53.2338) -> (10.0338, -53.2338)
  line L1130 (10.0338, -52.929) -> (10.0338, -53.2338)
  line L1131 (10.0338, -45.7662) -> (10.0338, -46.071)
  line L1132 (9.729, -45.7662) -> (10.0338, -45.7662)
  line L1133 (2.5662, -45.7662) -> (2.5662, -46.071)
  line L1134 (2.5662, -45.7662) -> (2.871, -45.7662)
  arc A170 (3.3282, -52.167) -> (3.9124, -52.167) centre (3.6203, -52.167) ccw
  arc A171 (3.9124, -52.167) -> (3.3282, -52.167) centre (3.6203, -52.167) ccw
  line L1135 (63.15, 51.6) -> (49.15, 51.6)
  line L1136 (49.15, 51.6) -> (49.15, 37.6)
  line L1137 (63.15, 37.6) -> (63.15, 51.6)
  line L1138 (49.15, 37.6) -> (63.15, 37.6)
  line L1139 (-9.8, -94.346) -> (-9.8, -87.854)
  arc A172 (-9.8, -87.854) -> (-10.054, -87.6) centre (-10.054, -87.854) ccw
  line L1140 (-10.054, -87.6) -> (-16.546, -87.6)
  arc A173 (-16.546, -87.6) -> (-16.8, -87.854) centre (-16.546, -87.854) ccw
  line L1141 (-16.8, -87.854) -> (-16.8, -94.346)
  arc A174 (-16.8, -94.346) -> (-16.546, -94.6) centre (-16.546, -94.346) ccw
  line L1142 (-16.546, -94.6) -> (-10.054, -94.6)
  arc A175 (-10.054, -94.6) -> (-9.8, -94.346) centre (-10.054, -94.346) ccw
  line L1143 (-14.44, -94.24) -> (-14.44, -87.96)
  line L1144 (3.4, -102.446) -> (3.4, -95.954)
  arc A176 (3.4, -95.954) -> (3.146, -95.7) centre (3.146, -95.954) ccw
  line L1145 (3.146, -95.7) -> (-3.346, -95.7)
  arc A177 (-3.346, -95.7) -> (-3.6, -95.954) centre (-3.346, -95.954) ccw
  line L1146 (-3.6, -95.954) -> (-3.6, -102.446)
  arc A178 (-3.6, -102.446) -> (-3.346, -102.7) centre (-3.346, -102.446) ccw
  line L1147 (-3.346, -102.7) -> (3.146, -102.7)
  arc A179 (3.146, -102.7) -> (3.4, -102.446) centre (3.146, -102.446) ccw
  line L1148 (-1.24, -102.34) -> (-1.24, -96.06)
  line L1149 (-22.346, -117.25) -> (-17.854, -117.25)
  arc A180 (-17.854, -117.25) -> (-17.6, -116.996) centre (-17.854, -116.996) ccw
  line L1150 (-17.6, -116.996) -> (-17.6, -112.204)
  arc A181 (-17.6, -112.204) -> (-17.854, -111.95) centre (-17.854, -112.204) ccw
  line L1151 (-17.854, -111.95) -> (-22.346, -111.95)
  arc A182 (-22.346, -111.95) -> (-22.6, -112.204) centre (-22.346, -112.204) ccw
  line L1152 (-22.6, -112.204) -> (-22.6, -116.996)
  arc A183 (-22.6, -116.996) -> (-22.346, -117.25) centre (-22.346, -116.996) ccw
  line L1153 (-22.24, -113.76) -> (-17.96, -113.76)
  line L1154 (20.2, -87.75) -> (20.2, -85.25)
  line L1155 (17, -85.25) -> (17, -87.75)
  line L1156 (17, -87.75) -> (20.2, -87.75)
  line L1157 (20.2, -85.25) -> (17, -85.25)
  line L1158 (20.2, -80.15) -> (20.2, -77.65)
  line L1159 (17, -77.65) -> (17, -80.15)
  line L1160 (17, -80.15) -> (20.2, -80.15)
  line L1161 (20.2, -77.65) -> (17, -77.65)
  line L1162 (3.6, -85.25) -> (3.6, -87.75)
  line L1163 (6.8, -87.75) -> (6.8, -85.25)
  line L1164 (6.8, -85.25) -> (3.6, -85.25)
  line L1165 (3.6, -87.75) -> (6.8, -87.75)
  line L1166 (3.6, -77.65) -> (3.6, -80.15)
  line L1167 (6.8, -80.15) -> (6.8, -77.65)
  line L1168 (6.8, -77.65) -> (3.6, -77.65)
  line L1169 (3.6, -80.15) -> (6.8, -80.15)
  line L1170 (15.9, -89.85) -> (15.9, -87.35)
  line L1171 (12.7, -87.35) -> (12.7, -89.85)
  line L1172 (12.7, -89.85) -> (15.9, -89.85)
  line L1173 (15.9, -87.35) -> (12.7, -87.35)
  line L1174 (4.6, -112.2) -> (4.6, -116.2)
  line L1175 (4.6, -116.2) -> (8.6, -116.2)
  line L1176 (8.6, -116.2) -> (8.6, -112.2)
  line L1177 (8.6, -112.2) -> (4.6, -112.2)
  line L1178 (4.96, -113.76) -> (8.34, -113.76)
  line L1179 (10.9, -95.7) -> (6.9, -95.7)
  line L1180 (6.9, -95.7) -> (6.9, -99.7)
  line L1181 (6.9, -99.7) -> (10.9, -99.7)
  line L1182 (10.9, -99.7) -> (10.9, -95.7)
  line L1183 (9.34, -96.06) -> (9.34, -99.44)
  line L1184 (-9.3, -113) -> (-9.3, -117)
  line L1185 (-9.3, -117) -> (-5.3, -117)
  line L1186 (-5.3, -117) -> (-5.3, -113)
  line L1187 (-5.3, -113) -> (-9.3, -113)
  line L1188 (-8.94, -114.56) -> (-5.56, -114.56)
  line L1189 (-6.2, 47.6) -> (-4.2, 47.6)
  line L1190 (-4.2, 47.6) -> (-4.2, 49.2)
  line L1191 (-6.2, 49.2) -> (-6.2, 47.6)
  line L1192 (-4.2, 49.2) -> (-6.2, 49.2)
  line L1193 (-7.1, 34.9) -> (-5.1, 34.9)
  line L1194 (-5.1, 34.9) -> (-5.1, 36.5)
  line L1195 (-7.1, 36.5) -> (-7.1, 34.9)
  line L1196 (-5.1, 36.5) -> (-7.1, 36.5)
  line L1197 (-0.2, 41) -> (-0.2, 43)
  line L1198 (-0.2, 43) -> (-1.8, 43)
  line L1199 (-1.8, 41) -> (-0.2, 41)
  line L1200 (-1.8, 43) -> (-1.8, 41)
  line L1201 (-9.025, -86.0924) -> (-10.9554, -86.0924)
  line L1202 (-15.375, -80.7076) -> (-12.5302, -80.7076)
  line L1203 (-10.9554, -80.7076) -> (-9.025, -80.7076)
  line L1204 (-12.5302, -86.0924) -> (-15.375, -86.0924)
  arc A184 (-8.4408, -81.876) -> (-8.4408, -81.114) centre (-8.3839, -81.495) ccw
  line L1205 (-9.3924, -96.575) -> (-9.3924, -94.6446)
  line L1206 (-4.0076, -90.225) -> (-4.0076, -93.0698)
  line L1207 (-4.0076, -94.6446) -> (-4.0076, -96.575)
  line L1208 (-9.3924, -93.0698) -> (-9.3924, -90.225)
  arc A185 (-5.176, -97.1592) -> (-4.414, -97.1592) centre (-4.795, -97.2161) ccw
  line L1209 (-9.3924, -103.375) -> (-9.3924, -101.4446)
  line L1210 (-4.0076, -97.025) -> (-4.0076, -99.8698)
  line L1211 (-4.0076, -101.4446) -> (-4.0076, -103.375)
  line L1212 (-9.3924, -99.8698) -> (-9.3924, -97.025)
  arc A186 (-5.176, -103.9592) -> (-4.414, -103.9592) centre (-4.795, -104.0161) ccw
  line L1213 (-6.75, 48.95) -> (-6.75, 52.25)
  line L1214 (-10.05, 52.25) -> (-10.05, 48.95)
  line L1215 (-10.05, 48.95) -> (-6.75, 48.95)
  line L1216 (-6.75, 52.25) -> (-10.05, 52.25)
  circle A187 centre (-9.15, 49.3) radius 0.1
  line L1217 (-14.925, 56.25) -> (-14.275, 56.25)
  line L1218 (-14.275, 57.95) -> (-14.925, 57.95)
  line L1219 (-14.275, 56.25) -> (-14.275, 56.682)
  line L1220 (-15.125, 57.152) -> (-15.125, 57.048)
  line L1221 (-14.275, 57.518) -> (-14.275, 57.95)
  line L1222 (-16.95, -21.225) -> (-16.95, -20.575)
  line L1223 (-18.65, -20.575) -> (-18.65, -21.225)
  line L1224 (-16.95, -20.575) -> (-17.382, -20.575)
  line L1225 (-17.852, -21.425) -> (-17.748, -21.425)
  line L1226 (-18.218, -20.575) -> (-18.65, -20.575)
  line L1227 (-18.85, -21.225) -> (-18.85, -20.575)
  line L1228 (-20.55, -20.575) -> (-20.55, -21.225)
  line L1229 (-18.85, -20.575) -> (-19.282, -20.575)
  line L1230 (-19.752, -21.425) -> (-19.648, -21.425)
  line L1231 (-20.118, -20.575) -> (-20.55, -20.575)
  line L1232 (-16.075, -40.75) -> (-16.725, -40.75)
  line L1233 (-16.725, -42.45) -> (-16.075, -42.45)
  line L1234 (-16.725, -40.75) -> (-16.725, -41.182)
  line L1235 (-15.875, -41.652) -> (-15.875, -41.548)
  line L1236 (-16.725, -42.018) -> (-16.725, -42.45)
  line L1237 (-7.075, -40.65) -> (-7.725, -40.65)
  line L1238 (-7.725, -42.35) -> (-7.075, -42.35)
  line L1239 (-7.725, -40.65) -> (-7.725, -41.082)
  line L1240 (-6.875, -41.552) -> (-6.875, -41.448)
  line L1241 (-7.725, -41.918) -> (-7.725, -42.35)
  line L1242 (17.125, -37.25) -> (16.475, -37.25)